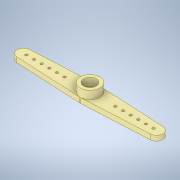
# Autodesk Inventor part: horn
Saved by Autodesk Inventor 2021 (Build 250183000, 183)
## iProperties
Created: 2016-07-11
Part Number: horn
Material: Nylon 6/6
Document SubType Name: Modeling
Designer: Diego
Density: 1.13 g/cm^3
Appearance: Nylon 6
Author: Diego
Autodesk Inventor part; units mm, degrees
ref_plane "YZ Plane" through (0, 0, 0) normal (1, 0, 0) x (0, 1, 0)
ref_plane "XZ Plane" through (0, 0, 0) normal (0, 1, 0) x (-1, 0, 0)
ref_plane "XY Plane" through (0, 0, 0) normal (0, 0, 1) x (1, 0, 0)
sketch "Sketch1" plane through (0, 0, 0) normal (0, 1, 0) x (-1, 0, 0)
  circle A0 centre (0, 0) radius 2.921
  circle A1 centre (0, 0) radius 1.905
  circle A2 centre (0, 0) radius 1
  line L0 (0.1488, 2.9172) -> (20.0361, 1.9025)
  circle A3 centre (19.939, 0) radius 1.905
  line L1 (0, 0) -> (0, 21.9223) construction
  line L2 (20.0361, -1.9025) -> (0.1488, -2.9172)
  line L3 (-0.1488, 2.9172) -> (-20.0361, 1.9025)
  circle A4 centre (-19.939, 0) radius 1.905
  line L4 (-20.0361, -1.9025) -> (-0.1488, -2.9172)
  line L5 (23.8294, 0) -> (-23.4157, 0) construction
  point P0 (19.05, 0)
  point P1 (16.764, 0)
  point P2 (14.478, 0)
  point P3 (12.192, 0)
  point P4 (9.906, 0)
  point P5 (7.62, 0)
  point P6 (-19.05, 0)
  point P7 (-16.764, 0)
  point P8 (-14.478, 0)
  point P9 (-12.192, 0)
  point P10 (-9.906, 0)
  point P11 (-7.62, 0)
  dimension "d0" = 5.842
  dimension "d1" = 3.81
  dimension "d2" = 2
  dimension "d3" = 43.688
  dimension "d4" = 3.81
  dimension "d11" = 2.286
  dimension "d16" = 38.1
  constraints: 12 end point, 9 symmetric about line, 8 point on circle, 6 tangent, 5 centre point, 3 coincident, 2 horizontal, 2 point on line, 1 horizontal alignment, 1 vertical, 6 other
  measures "d0" diameter of A0
  measures "d1" diameter of A1
  measures "d2" diameter of A2
  measures "d4" diameter of A3
  measures "d11" distance of point (19.05, 0) point (16.764, 0)
  measures "d16" distance of point (-19.05, 0) point (19.05, 0)
extrude "Extrusion1" add sketch "Sketch1" along normal blind 1.524 contours A0 | A0 L0 A3 L2 | A0 L4 A4 L3 | A3 | A4 | A1
extrude "Extrusion2" add sketch "Sketch1" along normal blind 3.937 contours A0
hole "Hole1" at (-19.05, 0, 0) at (-16.764, 0, 0) at (-14.478, 0, 0) at (-12.192, 0, 0) at (-9.906, 0, 0) at (-7.62, 0, 0) at (7.62, 0, 0) at (9.906, 0, 0) at (12.192, 0, 0) at (14.478, 0, 0) at (16.764, 0, 0) at (19.05, 0, 0) direction (0, 1, 0) diameter 0.762 end through all
extrude "Extrusion3" cut sketch "Sketch1" along normal blind 0.508 contours A1
body "Solid1"
